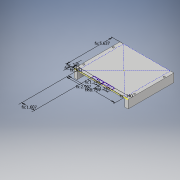
# Autodesk Inventor part: RioCoverPlate
Saved by Autodesk Inventor 2017 SP1 (Build 210196100, 196)
## iProperties
Created: 2016-11-23
Part Number: RioCoverPlate
Material: Generic
Document SubType Name: Modeling
Designer: steele
Density: 1 g/cm^3
Appearance: Default
Author: steele
Autodesk Inventor part; units mm, degrees
ref_plane "YZ Plane" through (0, 0, 0) normal (1, 0, 0) x (0, 1, 0)
ref_plane "XZ Plane" through (0, 0, 0) normal (0, 1, 0) x (-1, 0, 0)
ref_plane "XY Plane" through (0, 0, 0) normal (0, 0, 1) x (1, 0, 0)
sketch "Sketch1" plane through (0, 0, 0) normal (0, 0, 1) x (1, 0, 0)
  line L0 (0, 26.035) -> (-84.1883, 26.035)
  line L1 (-84.1883, 26.035) -> (-84.1883, 0)
  line L2 (-84.1883, 0) -> (-74.6633, 0)
  line L3 (-74.6633, 0) -> (-74.6633, 22.86)
  line L4 (-74.6633, 22.86) -> (0, 22.86)
  line L5 (0, 0) -> (0, 26.035) construction
  line L6 (0, 26.035) -> (84.1883, 26.035)
  line L7 (84.1883, 26.035) -> (84.1883, 0)
  line L8 (84.1883, 0) -> (74.6633, 0)
  line L9 (74.6633, 0) -> (74.6633, 22.86)
  line L10 (74.6633, 22.86) -> (0, 22.86)
  dimension "d0" = 22.86
  dimension "d1" = 3.175
  dimension "d2" = 9.525
  dimension "d3" = 74.6633
  constraints: 22 end point, 4 perpendicular, 4 symmetric about line, 1 horizontal, 1 vertical
  measures "d0" distance from line of L4 L5.start
  measures "d1" distance between parallel lines of L0 L4
  measures "d2" distance of L1.end L2.end
  measures "d3" distance of L2.end L5.start
extrude "Extrusion1" add sketch "Sketch1" along normal mid plane 143.1798
sketch "Sketch2" plane through (-84.1883, 0, 71.5899) normal (0, -1, 0) x (1, 0, 0)
  line L0 (0, -143.1798) -> (168.3766, -143.1798) construction
  line L1 (4.7625, -143.1798) -> (4.7625, -0.1575) construction
  line L2 (0, 0) -> (9.525, 0) projected
  point P0 (84.1883, -71.5899)
  point P1 (4.7625, -117.7798)
  point P2 (4.7625, -25.4)
  dimension "d6" = 4.7625
  dimension "d7" = 25.4
  dimension "d8" = 25.4
  constraints: 3 point on line, 2 end point, 1 vertical
  measures "d6" distance of L0.start L1.start
  measures "d7" distance of point (4.763, -117.78) L1.start
  measures "d8" distance from line of point (4.763, -25.4) L2
hole "Hole1" at (-79.4258, 0, -46.1899) at (-79.4258, 0, 46.1899) direction (0, 1, 0) diameter 5.1054 end through all clearance for "Flat Head Machine Screw (82)" size "#10" standard "Ansi Unified Screw Threads"
mirror "Mirror1" about plane through (0, 0, 0) normal (1, 0, 0) of "Hole1"
sketch "Sketch3" plane through (-84.1883, 26.035, 71.5899) normal (0, 1, 0) x (1, 0, 0)
  line L0 (11.1125, 0) -> (157.2641, 0) construction
  line L1 (157.2641, 0) -> (157.2641, 143.1798) construction
  line L2 (157.2641, 143.1798) -> (11.1125, 143.1798) construction
  line L3 (11.1125, 143.1798) -> (11.1125, 0) construction
  line L4 (11.1125, 0) -> (157.2641, 143.1798) construction
  line L5 (157.2641, 0) -> (11.1125, 143.1798) construction
  line L6 (51.9303, 1.2954) -> (83.4263, 1.2954)
  line L7 (83.4263, 1.2954) -> (83.4263, 9.9314)
  line L8 (83.4263, 9.9314) -> (51.9303, 9.9314)
  line L9 (51.9303, 9.9314) -> (51.9303, 1.2954)
  line L10 (51.9303, 1.2954) -> (83.4263, 9.9314) construction
  line L11 (83.4263, 1.2954) -> (51.9303, 9.9314) construction
  line L12 (168.3766, 0) -> (0, 0) projected
  line L13 (84.9503, 1.2954) -> (116.4463, 1.2954)
  line L14 (116.4463, 1.2954) -> (116.4463, 9.9314)
  line L15 (116.4463, 9.9314) -> (84.9503, 9.9314)
  line L16 (84.9503, 9.9314) -> (84.9503, 1.2954)
  line L17 (84.9503, 1.2954) -> (116.4463, 9.9314) construction
  line L18 (116.4463, 1.2954) -> (84.9503, 9.9314) construction
  point P0 (84.1883, 71.5899)
  point P1 (67.6783, 5.6134)
  point P2 (100.6983, 5.6134)
  dimension "d16" = 143.1798
  dimension "d17" = 146.1516
  dimension "d18" = 31.496
  dimension "d19" = 8.636
  dimension "d20" = 40.8178
  dimension "d21" = 1.2954
  dimension "d22" = 31.496
  dimension "d23" = 8.636
  dimension "d24" = 73.8378
  dimension "d25" = 1.2954
  constraints: 36 end point, 8 parallel, 6 midpoint, 3 perpendicular, 1 horizontal
  measures "d16" distance of L2.end L0.start
  measures "d17" distance of L0.start L0.end
  measures "d18" distance of L6.start L6.end
  measures "d19" distance of L8.end L6.start
  measures "d20" distance between parallel lines of L3 L9
  measures "d21" distance between parallel lines of L0 L6
  measures "d22" distance of L13.start L13.end
  measures "d23" distance of L13.end L14.end
  measures "d24" distance between parallel lines of L16 L3
  measures "d25" distance between parallel lines of L12 L13
equation "\"d0\" = heightForRIO"
equation "\"d1\" = topWallThickness"
equation "\"d2\" = edgeWallThickness"
equation "\"d3\" = 0.5 * widthOfRIO + widthAirGap"
equation "\"d4\" = depthOfRIO"
equation "\"d6\" = 0.5 * edgeWallThickness"
equation "\"d16\" = depthOfRIO"
equation "\"d17\" = widthOfRIO"
equation "\"d18\" = widthForBottomRelay"
equation "\"d19\" = depthForBottomRelay"
equation "\"d20\" = edgeToBottomRelay"
equation "\"d21\" = bottomToBottomRelay"
equation "\"d22\" = widthForBottomAnalogIn"
equation "\"d23\" = depthForBottomAnalogIn"
equation "\"d24\" = edgeToBottomAnalogIn"
equation "\"d25\" = bottomToBottomAnalogIn"
equation "\"heightForRIO\" = 22.86"
equation "\"topWallThickness\" = 3.175"
equation "\"edgeWallThickness\" = 9.525"
equation "\"widthOfRIO\" = 146.1516"
equation "\"widthAirGap\" = 1.5875"
equation "\"depthOfRIO\" = 143.1798"
equation "\"depthForBottomRelay\" = 8.636"
equation "\"widthForBottomRelay\" = 31.496"
equation "\"componentGap\" = 3.175"
equation "\"edgeToBottomRelay\" = 40.8178"
equation "\"bottomToBottomRelay\" = 1.2954"
equation "\"depthForBottomAnalogIn\" = 8.636"
equation "\"widthForBottomAnalogIn\" = 31.496"
equation "\"edgeToBottomAnalogIn\" = 73.8378"
equation "\"bottomToBottomAnalogIn\" = 1.2954"
body "Solid1"
